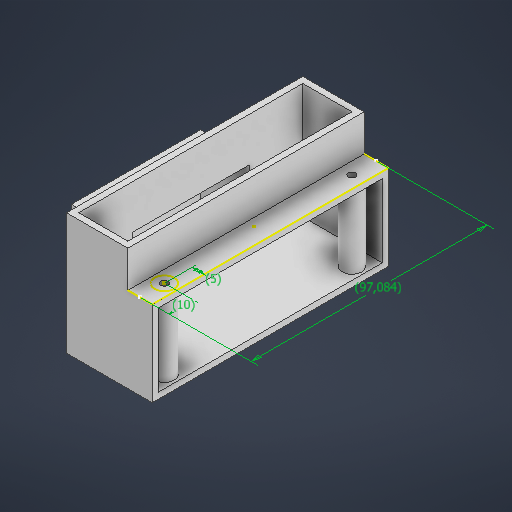
# Autodesk Inventor part: Sr. Batata
Saved by Autodesk Inventor 2026.1 (Build 301233020, 233B)
## iProperties
Created: 2025-11-07
Part Number: Sr. Batata
Material: Genérico
Document SubType Name: Modeling
Designer: david
Density: 1 g/cm^3
Appearance: Padrão
Author: david
Autodesk Inventor part; units mm, degrees
ref_plane "YZ Plane" through (0, 0, 0) normal (1, 0, 0) x (0, 1, 0)
ref_plane "XZ Plane" through (0, 0, 0) normal (0, 1, 0) x (-1, 0, 0)
ref_plane "XY Plane" through (0, 0, 0) normal (0, 0, 1) x (1, 0, 0)
sketch "Esboço1" plane through (0, 0, 0) normal (0, 1, 0) x (-1, 0, 0)
  line L0 (50, 50) -> (-50, 50)
  line L1 (-50, 50) -> (-50, -50)
  line L2 (-50, -50) -> (50, -50)
  line L3 (50, -50) -> (50, 50)
  line L4 (50, 50) -> (-50, -50) construction
  line L5 (-50, 50) -> (50, -50) construction
  line L6 (48.5421, 48.5421) -> (-6.6854, 48.5421)
  line L7 (-6.6854, 48.5421) -> (-6.6854, -48.542)
  line L8 (-6.6854, -48.542) -> (48.5421, -48.542)
  line L9 (48.5421, -48.542) -> (48.5421, 48.5421)
  line L10 (-6.6854, 48.5421) -> (3.3146, 48.5421)
  line L11 (3.3146, 48.5421) -> (3.3146, -48.542)
  line L12 (-1.6854, 48.5421) -> (8.3146, 48.5421)
  line L13 (-6.6854, 48.5421) -> (-1.6854, 48.5421)
  line L14 (-1.6854, 48.5421) -> (-1.6854, 38.5421)
  line L15 (-1.6854, 48.5421) -> (8.3146, 48.5421) construction
  circle A0 centre (-1.6854, 38.5421) radius 1.5
  line L16 (-6.6854, -48.542) -> (-1.6854, -48.542)
  line L17 (-1.6854, -48.542) -> (-1.6854, -38.542)
  circle A1 centre (-1.6854, -38.542) radius 1.5
  line L18 (48.5421, 0.0001) -> (28.5421, 0.0001)
  line L19 (28.5421, 48.5421) -> (28.5421, 26.5421)
  line L20 (28.5421, 26.5421) -> (48.5421, 26.5421)
  line L21 (28.5421, -48.542) -> (28.5421, -26.542)
  line L22 (28.5421, -48.542) -> (50.5421, -48.542) construction
  line L23 (28.5421, -26.542) -> (48.5421, -26.542)
  line L24 (28.5421, 26.5421) -> (28.5421, -26.542)
  point P0 (0, 0)
  dimension "d0" = 100
  dimension "d1" = 100
  dimension "d2" = 1.4579
  dimension "d3" = 1.458
  dimension "d4" = 43.3146
  dimension "d5" = 97.0841
  dimension "d6" = 10
  dimension "d7" = 10
  dimension "d8" = 5
  dimension "d9" = 10
  dimension "d10" = 90
  dimension "d11" = 3
  dimension "d12" = 5
  dimension "d13" = 10
  dimension "d14" = 90
  dimension "d15" = 3
  dimension "d16" = 55.2275
  dimension "d17" = 20
  dimension "d18" = 22
  dimension "d19" = 22
  dimension "d20" = 90
  dimension "d21" = 26.542
  constraints: 50 end point, 10 point on line, 9 perpendicular, 6 horizontal, 4 midpoint, 4 parallel, 2 centre point, 2 coincident, 2 vertical, 1 collinear
  measures "d0" distance of L2.end L1.end
  measures "d1" distance of L1.end L0.end
  measures "d2" distance between parallel lines of L6 L0
  measures "d3" distance between parallel lines of L2 L8
  measures "d4" distance between parallel lines of L1 L7
  measures "d5" distance between parallel lines of L8 L6
  measures "d6" distance of L6.end L10.end
  measures "d7" distance of L12.start L12.end
  measures "d8" distance of L6.end L12.start
  measures "d9" distance of L12.start L14.end
  measures "d10" angle of L14 L15
  measures "d11" diameter of A0
  measures "d12" distance of L7.end L16.end
  measures "d13" distance of L16.end L17.end
  measures "d14" angle of L17 L16
  measures "d15" diameter of A1
  measures "d16" distance between parallel lines of L7 L9
  measures "d17" distance of L18.start L18.end
  measures "d18" distance of L19.start L19.end
  measures "d19" distance of L21.start L21.end
  measures "d20" angle of L22 L21
  measures "d21" distance of L18.end L19.end
extrude "Extrusão1" add sketch "Esboço1" along normal blind 50 contours L19 L24 L21 L8 L11 L6
extrude "Extrusão2" add sketch "Esboço1" along normal blind 35 contours L11 L8 L7 L6
extrude "Extrusão3" add sketch "Esboço1" along normal blind 32 contours L9 L18 L24 L20 | L9 L23 L24 L18
thread "Rosca1" size "M3x0.5" class "6H" standard "ANSI Metric M Profile" length 20
thread "Rosca2" size "M3x0.5" class "6H" standard "ANSI Metric M Profile" length 20
shell "Casca1" thickness 2.5 removed faces 3 at (-35.2088, 32, -8.8473) at (-20.133, 50, 16.1807) at (6.6854, 11.6667, 16.1807)
sketch "Esboço2" plane through (0, 35, 0) normal (0, 1, 0) x (1, 0, 0)
  line L0 (-3.3146, -48.5421) -> (6.6854, -48.5421) projected
  line L1 (6.6854, 48.542) -> (-3.3146, 48.542) projected
  point P0 (0, 0)
  point P1 (1.6854, -48.5421)
  point P2 (1.6854, 48.542)
  dimension "d33" = 97.0841
  constraints: 2 midpoint
  measures "d33" distance of point (1.685, -48.542) point (1.685, 48.542)
sketch "Esboço3" plane through (0, 35, 0) normal (0, 1, 0) x (1, 0, 0)
  point P0 (0, 0)
sketch "Esboço4" plane through (0, 35, 0) normal (0, 1, 0) x (1, 0, 0)
  circle A0 centre (1.6854, -38.5421) radius 4 projected
  line L0 (-3.3146, -48.5421) -> (6.6854, -48.5421) projected
  line L1 (6.6854, -48.5421) -> (6.6854, 48.542) projected
  point P0 (0, 0)
  point P1 (1.6854, -48.5421)
  dimension "d34" = 10
  dimension "d35" = 5
  constraints: 1 midpoint
  measures "d34" distance of A0.centre point (1.685, -48.542)
  measures "d35" distance from line of L1 A0.centre
